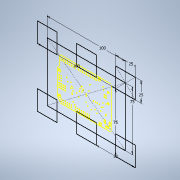
# Autodesk Inventor part: Base Para Arduino y Servos
Saved by Autodesk Inventor 2021 (Build 250183000, 183)
## iProperties
Created: 2021-02-17
Part Number: Base Para Arduino y Servos
Material: Generic
Document SubType Name: Modeling
Designer: Admin
Density: 1 g/cm^3
Appearance: Default
Author: Admin
Autodesk Inventor part; units mm, degrees
ref_plane "YZ Plane" through (0, 0, 0) normal (1, 0, 0) x (0, 1, 0)
ref_plane "XZ Plane" through (0, 0, 0) normal (0, 1, 0) x (-1, 0, 0)
ref_plane "XY Plane" through (0, 0, 0) normal (0, 0, 1) x (1, 0, 0)
sketch "Sketch1" plane through (0, 0, 0) normal (0, 0, 1) x (1, 0, 0)
  line L0 (-33.5997, -26.65) -> (30.4069, -26.65) projected
  line L1 (31.4013, -25.6555) -> (31.4013, 25.6344) projected
  line L2 (30.4069, 26.65) -> (-33.0707, 26.65) projected
  line L3 (31.4013, -25.6555) -> (31.4013, 25.6344) projected
  line L4 (31.359, -25.9094) -> (31.4013, -25.6555) projected
  line L5 (31.2744, -26.1422) -> (31.359, -25.9094) projected
  line L6 (31.1051, -26.3538) -> (31.2744, -26.1422) projected
  line L7 (30.8935, -26.523) -> (31.1051, -26.3538) projected
  line L8 (30.6608, -26.6077) -> (30.8935, -26.523) projected
  line L9 (30.4069, -26.65) -> (30.6608, -26.6077) projected
  line L10 (-33.5997, -26.65) -> (30.4069, -26.65) projected
  line L11 (-33.8536, -26.6077) -> (-33.5997, -26.65) projected
  line L12 (-34.0864, -26.523) -> (-33.8536, -26.6077) projected
  line L13 (-34.298, -26.3538) -> (-34.0864, -26.523) projected
  line L14 (-34.4672, -26.1422) -> (-34.298, -26.3538) projected
  line L15 (-34.5519, -25.9094) -> (-34.4672, -26.1422) projected
  line L16 (-34.5942, -25.6555) -> (-34.5519, -25.9094) projected
  line L17 (-34.5942, -24.1109) -> (-34.5942, -25.6555) projected
  line L18 (-37.1333, -21.5718) -> (-34.5942, -24.1109) projected
  line L19 (-37.1333, 11.1615) -> (-37.1333, -21.5718) projected
  line L20 (-34.5942, 13.7006) -> (-37.1333, 11.1615) projected
  line L21 (-34.5942, 25.1265) -> (-34.5942, 13.7006) projected
  line L22 (-33.0707, 26.65) -> (-34.5942, 25.1265) projected
  line L23 (30.4069, 26.65) -> (-33.0707, 26.65) projected
  line L24 (30.6608, 26.6077) -> (30.4069, 26.65) projected
  line L25 (30.8935, 26.5019) -> (30.6608, 26.6077) projected
  line L26 (31.1051, 26.3538) -> (30.8935, 26.5019) projected
  line L27 (31.2744, 26.1422) -> (31.1051, 26.3538) projected
  line L28 (31.359, 25.9094) -> (31.2744, 26.1422) projected
  line L29 (31.4013, 25.6344) -> (31.359, 25.9094) projected
  circle A0 centre (-29.5466, 23.876) radius 0.4445 projected
  circle A1 centre (-32.0866, 23.876) radius 0.4445 projected
  circle A2 centre (-32.0866, 21.336) radius 0.4445 projected
  circle A3 centre (-29.5466, 21.336) radius 0.4445 projected
  circle A4 centre (-27.0066, 21.336) radius 0.4445 projected
  circle A5 centre (-27.0066, 23.876) radius 0.4445 projected
  circle A6 centre (-24.4666, 23.876) radius 0.4445 projected
  circle A7 centre (-24.4666, 21.336) radius 0.4445 projected
  circle A8 centre (-21.9266, 23.876) radius 0.4445 projected
  circle A9 centre (-21.9266, 21.336) radius 0.4445 projected
  circle A10 centre (-14.3066, 21.336) radius 0.4445 projected
  circle A11 centre (-14.3066, 23.876) radius 0.4445 projected
  circle A12 centre (-16.8466, 23.876) radius 0.4445 projected
  circle A13 centre (-16.8466, 21.336) radius 0.4445 projected
  circle A14 centre (-19.3866, 21.336) radius 0.4445 projected
  circle A15 centre (-19.3866, 23.876) radius 0.4445 projected
  circle A16 centre (12.3634, 21.336) radius 0.4445 projected
  circle A17 centre (12.3634, 23.876) radius 0.4445 projected
  circle A18 centre (9.8234, 23.876) radius 0.4445 projected
  circle A19 centre (9.8234, 21.336) radius 0.4445 projected
  circle A20 centre (7.2834, 21.336) radius 0.4445 projected
  circle A21 centre (7.2834, 23.876) radius 0.4445 projected
  circle A22 centre (4.7434, 21.336) radius 0.4445 projected
  circle A23 centre (4.7434, 23.876) radius 0.4445 projected
  circle A24 centre (2.2034, 23.876) radius 0.4445 projected
  circle A25 centre (2.2034, 21.336) radius 0.4445 projected
  circle A26 centre (-0.3366, 21.336) radius 0.4445 projected
  circle A27 centre (-0.3366, 23.876) radius 0.4445 projected
  circle A28 centre (-2.8766, 23.876) radius 0.4445 projected
  circle A29 centre (-10.4966, 23.876) radius 0.4445 projected
  circle A30 centre (-7.9566, 23.876) radius 0.4445 projected
  circle A31 centre (-5.4166, 23.876) radius 0.4445 projected
  circle A32 centre (-2.8766, 21.336) radius 0.4445 projected
  circle A33 centre (-5.4166, 21.336) radius 0.4445 projected
  circle A34 centre (-7.9566, 21.336) radius 0.4445 projected
  circle A35 centre (-10.4966, 21.336) radius 0.4445 projected
  circle A36 centre (27.5454, 15.2603) radius 1.2 projected
  circle A37 centre (24.8353, 10.394) radius 0.55 projected
  circle A38 centre (22.8353, 10.394) radius 0.55 projected
  circle A39 centre (24.8353, 7.894) radius 0.55 projected
  circle A40 centre (22.8353, 7.894) radius 0.55 projected
  circle A41 centre (27.5454, 3.0277) radius 1.2 projected
  circle A42 centre (16.4274, -3.302) radius 0.4445 projected
  circle A43 centre (13.8874, -3.302) radius 0.4445 projected
  circle A44 centre (11.3474, -3.302) radius 0.4445 projected
  circle A45 centre (8.8074, -3.302) radius 0.4445 projected
  circle A46 centre (24.9618, -10.3124) radius 0.305 projected
  circle A47 centre (3.4734, -21.844) radius 0.4445 projected
  circle A48 centre (3.4734, -24.384) radius 0.4445 projected
  circle A49 centre (0.9334, -24.384) radius 0.4445 projected
  circle A50 centre (0.9334, -21.844) radius 0.4445 projected
  circle A51 centre (-1.6066, -21.844) radius 0.4445 projected
  circle A52 centre (-1.6066, -24.384) radius 0.4445 projected
  circle A53 centre (-4.1466, -24.384) radius 0.4445 projected
  circle A54 centre (-4.1466, -21.844) radius 0.4445 projected
  circle A55 centre (-6.6866, -24.384) radius 0.4445 projected
  circle A56 centre (-6.6866, -21.844) radius 0.4445 projected
  circle A57 centre (-9.2266, -21.844) radius 0.4445 projected
  circle A58 centre (-9.2266, -24.384) radius 0.4445 projected
  circle A59 centre (-11.7666, -24.384) radius 0.4445 projected
  circle A60 centre (-11.7666, -21.844) radius 0.4445 projected
  circle A61 centre (-14.3066, -21.844) radius 0.4445 projected
  circle A62 centre (-14.3066, -24.384) radius 0.4445 projected
  circle A63 centre (-29.5466, -24.384) radius 0.4445 projected
  circle A64 centre (-27.0066, -24.384) radius 0.4445 projected
  circle A65 centre (-24.4666, -24.384) radius 0.4445 projected
  circle A66 centre (-21.9266, -24.384) radius 0.4445 projected
  circle A67 centre (-19.3866, -24.384) radius 0.4445 projected
  circle A68 centre (-19.3866, -21.844) radius 0.4445 projected
  circle A69 centre (-21.9266, -21.844) radius 0.4445 projected
  circle A70 centre (-24.4666, -21.844) radius 0.4445 projected
  circle A71 centre (-27.0066, -21.844) radius 0.4445 projected
  circle A72 centre (-29.5466, -21.844) radius 0.4445 projected
  circle A73 centre (-32.0866, -21.844) radius 0.4445 projected
  circle A74 centre (-32.0866, -24.384) radius 0.4445 projected
  circle A75 centre (-29.8006, -7.62) radius 0.4445 projected
  circle A76 centre (-32.3406, -7.62) radius 0.4445 projected
  circle A77 centre (-34.8806, -7.62) radius 0.4445 projected
  circle A78 centre (-34.8806, -5.08) radius 0.4445 projected
  circle A79 centre (-32.3406, -5.08) radius 0.4445 projected
  circle A80 centre (-29.8006, -5.08) radius 0.4445 projected
  circle A81 centre (-27.2606, -5.08) radius 0.4445 projected
  circle A82 centre (-27.2606, -7.62) radius 0.4445 projected
  circle A83 centre (-27.2606, -10.16) radius 0.4445 projected
  circle A84 centre (-29.8006, -10.16) radius 0.4445 projected
  circle A85 centre (-32.3406, -10.16) radius 0.4445 projected
  circle A86 centre (-34.8806, -10.16) radius 0.4445 projected
  circle A87 centre (-32.2136, 3.683) radius 0.4445 projected
  circle A88 centre (-34.7536, 3.683) radius 0.4445 projected
  circle A89 centre (-34.7536, -1.397) radius 0.4445 projected
  circle A90 centre (-32.2136, -1.397) radius 0.4445 projected
  circle A91 centre (-32.2136, 1.143) radius 0.4445 projected
  circle A92 centre (-34.7536, 1.143) radius 0.4445 projected
  circle A93 centre (-9.0488, -1.7932) radius 0.305 projected
  circle A94 centre (21.0324, -4.5542) radius 0.305 projected
  line L30 (28.4332, -17.4319) -> (28.4332, -20.0319) projected
  arc A95 (28.4332, -20.0319) -> (30.4332, -20.0319) centre (29.4332, -20.0319) ccw projected
  line L31 (30.4332, -20.0319) -> (30.4332, -17.4319) projected
  arc A96 (30.4332, -17.4319) -> (28.4332, -17.4319) centre (29.4332, -17.4319) ccw projected
  line L32 (24.2335, -20.0319) -> (24.2335, -17.4319) projected
  arc A97 (24.2335, -17.4319) -> (22.2335, -17.4319) centre (23.2335, -17.4319) ccw projected
  line L33 (22.2335, -20.0319) -> (22.2335, -17.4319) projected
  arc A98 (22.2335, -20.0319) -> (24.2335, -20.0319) centre (23.2335, -20.0319) ccw projected
  circle A99 centre (-18.8583, -1.2548) radius 0.305 projected
  circle A100 centre (-24.1796, 1.4021) radius 0.305 projected
  circle A101 centre (-25.127, 5.522) radius 0.305 projected
  circle A102 centre (-0.3086, -0.4953) radius 0.305 projected
  circle A103 centre (-0.3086, -2.5908) radius 0.305 projected
  circle A104 centre (-0.5652, -9.525) radius 0.305 projected
  circle A105 centre (-4.3396, 1.5443) radius 0.305 projected
  circle A106 centre (1.7259, -12.4562) radius 0.305 projected
  circle A107 centre (-6.5672, 4.257) radius 0.305 projected
  circle A108 centre (-20.0317, -3.6195) radius 0.305 projected
  circle A109 centre (24.9237, 1.2344) radius 0.305 projected
  circle A110 centre (-17.2352, -5.5245) radius 0.305 projected
  circle A111 centre (-4.6165, 2.7203) radius 0.305 projected
  circle A112 centre (6.1861, -14.4069) radius 0.305 projected
  circle A113 centre (24.2938, -11.8237) radius 0.305 projected
  circle A114 centre (-8.2131, 1.5367) radius 0.305 projected
  circle A115 centre (-12.5413, -5.2019) radius 0.305 projected
  circle A116 centre (10.7759, -11.9939) radius 0.305 projected
  circle A117 centre (17.9768, -9.8984) radius 0.305 projected
  circle A118 centre (16.1734, 24.13) radius 1.75 projected
  circle A119 centre (17.4434, -24.13) radius 1.75 projected
  circle A120 centre (21.2204, 18.5141) radius 0.305 projected
  circle A121 centre (21.2204, 0.3962) radius 0.305 projected
  circle A122 centre (-18.5382, -8.3693) radius 0.305 projected
  circle A123 centre (-34.6266, -19.05) radius 1.75 projected
  circle A124 centre (-5.7239, -1.0033) radius 0.305 projected
  circle A125 centre (-15.1651, -19.718) radius 0.305 projected
  circle A126 centre (-17.0193, -17.2568) radius 0.305 projected
  circle A127 centre (13.4556, -14.7625) radius 0.305 projected
  arc A128 (24.9333, -22.4321) -> (24.9333, -24.4321) centre (24.9333, -23.4321) ccw projected
  line L34 (27.5333, -24.4321) -> (24.9333, -24.4321) projected
  arc A129 (27.5333, -24.4321) -> (27.5333, -22.4321) centre (27.5333, -23.4321) ccw projected
  line L35 (24.9333, -22.4321) -> (27.5333, -22.4321) projected
  circle A130 centre (3.0543, 4.6533) radius 0.305 projected
  circle A131 centre (-18.175, -9.7663) radius 0.305 projected
  circle A132 centre (-5.9424, 5.3365) radius 0.305 projected
  circle A133 centre (21.8732, 15.1587) radius 0.305 projected
  circle A134 centre (-9.854, -8.448) radius 0.305 projected
  circle A135 centre (-34.6266, 8.89) radius 1.75 projected
  circle A136 centre (4.3142, 12.1691) radius 0.305 projected
  circle A137 centre (18.9344, -5.2654) radius 0.305 projected
  circle A138 centre (-17.5781, -2.1971) radius 0.305 projected
  circle A139 centre (-19.7727, 2.7432) radius 0.305 projected
  line L36 (-50.3086, -45.4953) -> (49.6914, -45.4953)
  line L37 (49.6914, -45.4953) -> (49.6914, 44.5047)
  line L38 (49.6914, 44.5047) -> (-50.3086, 44.5047)
  line L39 (-50.3086, 44.5047) -> (-50.3086, -45.4953)
  line L40 (-50.3086, -45.4953) -> (37.1914, 33.2547) construction
  line L41 (37.1914, -34.2453) -> (-50.3086, 44.5047) construction
  line L42 (37.1914, 32.0047) -> (62.1914, 32.0047)
  line L43 (62.1914, 32.0047) -> (62.1914, 57.0047)
  line L44 (62.1914, 57.0047) -> (37.1914, 57.0047)
  line L45 (37.1914, 57.0047) -> (37.1914, 32.0047)
  line L46 (61.1149, 55.9283) -> (62.1914, 57.0047) construction
  line L47 (49.6914, 44.5047) -> (44.0436, 50.1525) construction
  line L48 (37.1914, -57.9953) -> (62.1914, -57.9953)
  line L49 (62.1914, -32.9953) -> (37.1914, -32.9953)
  line L50 (62.1914, -57.9953) -> (62.1914, -32.9953)
  line L51 (37.1914, -32.9953) -> (37.1914, -57.9953)
  line L52 (-62.8086, 32.0047) -> (-37.8086, 32.0047)
  line L53 (-37.8086, 57.0047) -> (-62.8086, 57.0047)
  line L54 (-37.8086, 32.0047) -> (-37.8086, 57.0047)
  line L55 (-62.8086, 57.0047) -> (-62.8086, 32.0047)
  line L56 (-62.8086, -57.9953) -> (-37.8086, -57.9953)
  line L57 (-37.8086, -32.9953) -> (-62.8086, -32.9953)
  line L58 (-37.8086, -57.9953) -> (-37.8086, -32.9953)
  line L59 (-62.8086, -32.9953) -> (-62.8086, -57.9953)
  line L60 (12.1914, -57.9953) -> (12.1914, -32.9953)
  line L61 (12.1914, -32.9953) -> (-12.8086, -32.9953)
  line L62 (-12.8086, -57.9953) -> (12.1914, -57.9953)
  line L63 (-12.8086, -32.9953) -> (-12.8086, -57.9953)
  line L64 (-12.8086, 57.0047) -> (-12.8086, 32.0047)
  line L65 (-12.8086, 32.0047) -> (12.1914, 32.0047)
  line L66 (12.1914, 32.0047) -> (12.1914, 57.0047)
  line L67 (12.1914, 57.0047) -> (-12.8086, 57.0047)
  arc A140 (62.1914, -32.9953) -> (62.1914, 32.0047) centre (38.8729, -0.4953) ccw
  arc A141 (-62.8086, 32.0047) -> (-62.8086, -32.9953) centre (-39.4902, -0.4953) ccw
  point P0 (0, 0)
  point P1 (-37.8086, 44.5047)
  point P2 (-37.8086, -45.4953)
  point P3 (-12.8086, -45.4953)
  point P4 (12.1914, -45.4953)
  point P5 (37.1914, -45.4953)
  point P6 (37.1914, 44.5047)
  point P7 (12.1914, 44.5047)
  point P8 (-12.8086, 44.5047)
  dimension "d0" = 100
  dimension "d1" = 90
  dimension "d2" = 25
  dimension "d3" = 25
  dimension "d6" = 90
  dimension "d9" = 100
  dimension "d14" = 50
  dimension "d19" = 40
  dimension "d20" = 40
  dimension "d21" = 0.3086
  constraints: 64 end point, 6 point on line, 4 horizontal, 4 parallel, 4 point on circle, 2 centre point, 2 perpendicular, 1 vertical, 40 other
  measures "d0" distance of L37.end L38.end
  measures "d1" distance of L37.end L36.end
  measures "d2" distance of L43.end L44.end
  measures "d3" distance of L42.end L43.end
  measures "d6" distance of L42.start L48.start
  measures "d9" distance of L42.start L52.start
  measures "d14" distance of L48.end L60.start
  measures "d19" radius of A140
  measures "d20" radius of A141
  measures "d21" horizontal distance of point (0, 0) A102.centre
extrude "Extrusion1" add sketch "Sketch1" along normal blind 10 contours L11 L12 L13 L14 L15 L16 L17 L18 L19 L20 L21 L22 L2 L24 L25 L26 L27 L28 L29 L1 L4 L5 L6 L7 L8 L9 L0 | L39 L57 L58 L36 | L36 L58 L56 L59 L57 L39 | L58 L57 L39 L52 L54 L38 L64 L65 L66 L45 L42 L37 L49 L51 L36 L60 L61 L63 | L57 A141 L52 L39 | L63 L61 L60 L36 | L36 L60 L62 L63 | L52 L55 L53 L54 L38 L39 | L39 L38 L54 L52 | L51 L49 L37 L36 | L36 L37 L49 L50 L48 L51 | L64 L67 L66 L38 | L38 L66 L65 L64 | L37 L42 A140 L49 | L42 L45 L38 L37 | L37 L38 L45 L44 L43 L42
body "Solid1"
